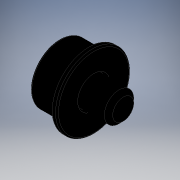
# Autodesk Inventor part: F682ZZ
Saved by Autodesk Inventor 2019 (Build 230136000, 136)
## iProperties
Created: 2024-06-28
Part Number: F682ZZ
Material: Generic
Catalog Web Link: www.cadenas.de
Description: MF63ZZ, F63ZZ, F685ZZ-Extra Small Bearings - Miniature Ball Bearings
Vendor: MISUMI
Document SubType Name: Modeling
Designer: psAdmin
Manufacturer: MISUMI
Mass: 0.0391275 g
Surface Area: 0.859263 cm^2
Volume: 0.0391275 cm^3
Density: 1 g/cm^3
Appearance: PSOLRGB-0-0-0
Category: PARTsolutions
Company: MISUMI
Title: F682ZZ
Author: Cadenas PARTsolutions
Comments: Extra Small Bearings - Miniature Ball Bearings
PSOL_IDENT_0: {$CADENAS_DATA/23d-libs/misumi/metric/07_slide_rails/bearing.prj},158 {VTYP=3D},{NB=F682ZZ},{LINA=F6
PSOL_IDENT_1: 82ZZ},{NN=MF63ZZ, F63ZZ, F685ZZ},{DATE=30.06.2021 12:53:44},{GEOMDATE=08.09.2006},{VERSION=},{LINEID=
PSOL_IDENT_2: 10},{WBVAR=},{WBNUMERIC=}  {NB=F682ZZ},{LINA=F682ZZ},{KT=DUMMY},{PN=F682ZZ},{TYPE=F682ZZ},{DD=2.0},{
PSOL_IDENT_3: D=4},{D2=5.0},{B1=2.5},{C2=0.42426},{RR1=0.1},{DMIN=1.567},{DMAX=2.000},{L=2.000},{D10=0.180}
NB: F682ZZ
NN: MF63ZZ, F63ZZ, F685ZZ
NT: Extra Small Bearings - Miniature Ball Bearings
NBSYN: $PN.
LINA: F682ZZ
CATALOG: Misumi
TYPE: F682ZZ
DD: 2
D: 4
D2: 5
B1: 2.5
C2: 0.42426
RR1: 0.1
DMIN: 1.567
DMAX: 2
L: 2
D10: 0.18
SUPPLIER: MISUMI
ARTICLENO: F682ZZ
BOMINFO: F682ZZ
CREATOR: CADENAS GmbH
Autodesk Inventor part; units mm, degrees
sketch "Sketch_1" plane through (0, 0, 0) normal (0, 0, 1) x (1, 0, 0)
  line L0 (2.32, 0) -> (0, 0)
  arc A0 (0, 1.1) -> (0.1, 1) centre (0.1, 1.1) ccw
  line L1 (0.1, 1) -> (2.22, 1)
  arc A1 (2.22, 1) -> (2.32, 1.1) centre (2.22, 1.1) ccw
  line L2 (2.32, 1.1) -> (2.32, 2.4)
  arc A2 (2.32, 2.4) -> (2.22, 2.5) centre (2.22, 2.4) ccw
  line L3 (2.22, 2.5) -> (1.9957, 2.5)
  arc A3 (1.9957, 2.5) -> (1.8957, 2.4) centre (1.9957, 2.4) ccw
  line L4 (1.8957, 2.4) -> (1.8957, 2.05)
  arc A4 (1.8457, 2) -> (1.8957, 2.05) centre (1.8957, 2) ccw
  line L5 (1.8457, 2) -> (0.1, 2)
  arc A5 (0.1, 2) -> (0, 1.9) centre (0.1, 1.9) ccw
  line L6 (0, 1.9) -> (0, 1.1)
  constraints: 14 end point, 12 point on circle, 6 centre point
revolve "Revolution1" add sketch "Sketch_1" angle 360 about axis through (2.32, 0, 0) along (1, 0, 0)
sketch "Sketch_3" plane through (0, 0, 0) normal (0, 1, 0) x (-1, 0, 0)
  line L0 (0.2, 0) -> (-4.32, 0)
  line L1 (-4.32, 0) -> (-4.32, 0.7151)
  line L2 (-4.32, 0.7151) -> (-4.0351, 1)
  line L3 (-4.0351, 1) -> (0, 1)
  line L4 (0, 1) -> (0, 1.3333)
  line L5 (0, 1.3333) -> (0.2, 1.3333)
  line L6 (0.2, 1.3333) -> (0.2, 0)
  line L7 (0.2, 0) -> (-4.32, 0)
  constraints: 16 end point
revolve "Revolution2" add sketch "Sketch_3" angle 360 about axis through (-0.2, 0, 0) along (-1, 0, 0)
ref_plane "to_block_XY" through (2.32, 0, 0) normal (1, 0, 0) x (0, 0, -1)
ref_plane "to_block_YZ" through (2.32, 0, 0) normal (0, 0, -1) x (0, 1, 0)
ref_plane "to_block_ZX" through (2.32, 0, 0) normal (0, 1, 0) x (1, 0, 0)
body "Solid1"
